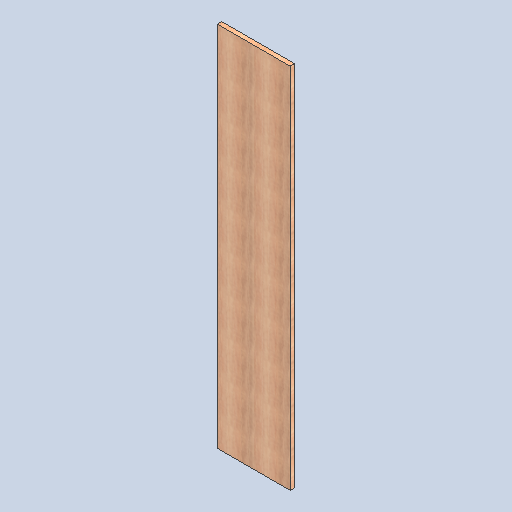
# Autodesk Inventor part: madeiraControladora
Saved by Autodesk Inventor 2025 (Build 290162000, 162)
## iProperties
Created: 2022-08-17
Part Number: madeiraControladora
Material: Generic
Document SubType Name: Modeling
Designer: cvss2
Density: 1 g/cm^3
Appearance: Default
Author: cvss2
Autodesk Inventor part; units mm, degrees
ref_plane "YZ Plane" through (0, 0, 0) normal (1, 0, 0) x (0, 1, 0)
ref_plane "XZ Plane" through (0, 0, 0) normal (0, 1, 0) x (-1, 0, 0)
ref_plane "XY Plane" through (0, 0, 0) normal (0, 0, 1) x (1, 0, 0)
sketch "Sketch1" plane through (0, 0, 0) normal (0, 0, 1) x (1, 0, 0)
  line L0 (0, 0) -> (-494, 0)
  line L1 (-494, 0) -> (-494, -2494)
  line L2 (-494, -2494) -> (0, -2494)
  line L3 (0, -2494) -> (0, 0)
  dimension "d0" = 494
  dimension "d1" = 2494
  constraints: 8 end point, 2 parallel, 1 horizontal, 1 perpendicular
  measures "d0" distance of L2.end L1.end
  measures "d1" distance of L1.end L0.end
extrude "Extrusion1" add sketch "Sketch1" along normal blind 30
body "Solid1"
